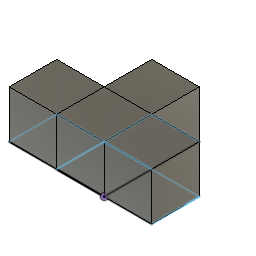
BooleanOverlap3Way (Autodesk Fusion 360 design; units mm, degrees)
Autodesk Fusion 360 part; units mm, degrees
sketch "Sketch1" plane through (0, 0, 0) normal (0, 0, 1) x (1, 0, 0)
  line L0 (0, 0) -> (-10, 0)
  line L1 (-10, 0) -> (-10, 20)
  line L2 (-10, 20) -> (0, 20)
  line L3 (0, 20) -> (0, 0)
  line L4 (0, 0) -> (-20, 0)
  line L5 (-20, 0) -> (-20, 10)
  line L6 (-20, 10) -> (0, 10)
  line L7 (0, 10) -> (0, 0)
  line L8 (-10, 0) -> (10, 0)
  line L9 (10, 0) -> (10, 10)
  line L10 (10, 10) -> (-10, 10)
  line L11 (-10, 10) -> (-10, 0)
  constraint horizontal L0
  constraint vertical L1
  constraint horizontal L2
  constraint vertical L3
  constraint coincident L0.start L3.end
  constraint horizontal L4
  constraint vertical L5
  constraint horizontal L6
  constraint vertical L7
  constraint horizontal L8
  constraint vertical L9
  constraint horizontal L10
  constraint vertical L11
extrude "Extrude1" add sketch "Sketch1" along normal blind 10 contours L0 L1 L3 L4 L6 L7 L8 L10 L11 | L1 L4 L5 L6 L11 makes body 1
extrude "Extrude2" add sketch "Sketch1" along normal blind 10 separate body contours L0 L1 L3 L4 L6 L7 L8 L10 L11 | L1 L2 L3 L6 L10 makes body 2
extrude "Extrude3" add sketch "Sketch1" along normal blind 10 separate body contours L0 L1 L3 L4 L6 L7 L8 L10 L11 | L3 L7 L8 L9 L10 makes body 3
